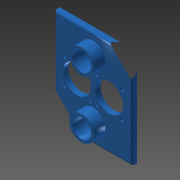
# Autodesk Inventor part: XCarriageV9Top
Saved by Autodesk Inventor 2015 (Build 190159000, 159)
## iProperties
Created: 2014-08-22
Part Number: XCarriageV9Top
Material: ABS Plastic
Document SubType Name: Modeling
Designer: Jack
Density: 1.06 g/cm^3
Appearance: Cyan
Author: Jack
Autodesk Inventor part; units mm, degrees
ref_plane "YZ Plane" through (0, 0, 0) normal (1, 0, 0) x (0, 1, 0)
ref_plane "XZ Plane" through (0, 0, 0) normal (0, 1, 0) x (-1, 0, 0)
ref_plane "XY Plane" through (0, 0, 0) normal (0, 0, 1) x (1, 0, 0)
sketch "Sketch1" plane through (0, 0, 0) normal (0, 1, 0) x (-1, 0, 0)
  line L0 (0, 0) -> (72, 0)
  line L1 (72, 0) -> (72, -90)
  line L2 (72, -90) -> (0, -90)
  line L3 (0, -90) -> (0, 0)
  dimension "d0" = 72
  dimension "d1" = 90
  constraints: 8 end point, 2 parallel, 1 horizontal, 1 perpendicular
  measures "d0" distance of L0.start L0.end
  measures "d1" distance of L2.end L0.start
extrude "Extrusion1" add sketch "Sketch1" along normal blind 5
sketch "Sketch2" plane through (0, 0, 0) normal (0, -1, 0) x (1, 0, 0)
  line L0 (-72, 0) -> (-72, -90) projected
  line L1 (-72, -90) -> (0, -90) projected
  circle A0 centre (-36, -72) radius 8.75
  circle A1 centre (-36, -18) radius 8.75
  circle A2 centre (-36, -18) radius 11.5
  circle A3 centre (-36, -72) radius 11.5
  dimension "d4" = 17.5
  dimension "d5" = 23
  dimension "d6" = 54
  dimension "d7" = 18
  dimension "d8" = 36
  constraints: 4 centre point, 2 coincident, 2 equal radius, 1 vertical alignment
  measures "d4" diameter of A1
  measures "d5" diameter of A2
  measures "d6" distance of A0.centre A1.centre
  measures "d7" distance from line of L1 A0.centre
  measures "d8" distance from line of L0 A0.centre
extrude "Extrusion2" add sketch "Sketch2" along normal blind 10.7
sketch "Sketch3" plane through (-36, 0, -18) normal (0, -1, 0) x (1, 0, 0)
  circle A0 centre (0, 0) radius 8.75 projected
  circle A1 centre (0, -54) radius 8.75 projected
  point P0 (36, 18)
extrude "Extrusion3" cut sketch "Sketch3" against normal up to surface (5 mm away)
sketch "Sketch4" plane through (0, 0, 0) normal (0, -1, 0) x (1, 0, 0)
  line L0 (0, 0) -> (-72, 0) projected
  line L1 (-72, 0) -> (-72, -90) projected
  line L2 (0, -90) -> (0, 0) projected
  circle A0 centre (-21, -45) radius 13
  circle A1 centre (-51, -45) radius 13
  dimension "d14" = 26
  dimension "d16" = 21
  dimension "d17" = 21
  dimension "d18" = 45
  constraints: 2 centre point, 1 equal radius, 1 horizontal alignment
  measures "d14" diameter of A1
  measures "d16" distance from line of L1 A1.centre
  measures "d17" distance from line of L2 A0.centre
  measures "d18" distance from line of L0 A0.centre
extrude "Extrusion4" cut sketch "Sketch4" against normal up to surface (5 mm away)
sketch "Sketch5" plane through (0, 0, 0) normal (0, -1, 0) x (1, 0, 0)
  circle A0 centre (-21, -45) radius 13 projected
  circle A1 centre (-51, -45) radius 13 projected
  circle A2 centre (-9, -57) radius 1.5
  circle A3 centre (-9, -33) radius 1.5
  circle A4 centre (-33, -57) radius 1.5
  circle A5 centre (-33, -33) radius 1.5
  circle A6 centre (-39, -33) radius 1.5
  circle A7 centre (-39, -57) radius 1.5
  circle A8 centre (-63, -57) radius 1.5
  circle A9 centre (-63, -33) radius 1.5
  dimension "d21" = 3
  dimension "d22" = 24
  dimension "d23" = 24
  dimension "d24" = 24
  dimension "d25" = 12
  dimension "d26" = 12
  dimension "d27" = 12
  constraints: 8 centre point, 7 equal radius, 6 horizontal alignment, 4 vertical alignment
  measures "d21" diameter of A2
  measures "d22" distance of A8.centre A7.centre
  measures "d23" distance of A2.centre A4.centre
  measures "d24" distance of A2.centre A3.centre
  measures "d25" horizontal distance of A0.centre A2.centre
  measures "d26" horizontal distance of A0.centre A2.centre
  measures "d27" horizontal distance of A1.centre A7.centre
extrude "Extrusion5" cut sketch "Sketch5" against normal up to surface (5 mm away) contours A2 | A3 | A4 | A5 | A6 | A7 | A8 | A9
sketch "Sketch6" plane through (0, 5, 0) normal (0, 1, 0) x (1, 0, 0)
  circle A0 centre (-39, 57) radius 1.5 projected
  circle A1 centre (-33, 33) radius 1.5 projected
  circle A2 centre (-33, 57) radius 1.5 projected
  circle A3 centre (-39, 33) radius 1.5 projected
  line L0 (-39, 60.1754) -> (-36.25, 58.5877)
  line L1 (-36.25, 58.5877) -> (-36.25, 55.4123)
  line L2 (-36.25, 55.4123) -> (-39, 53.8246)
  line L3 (-39, 53.8246) -> (-41.75, 55.4123)
  line L4 (-41.75, 55.4123) -> (-41.75, 58.5877)
  line L5 (-41.75, 58.5877) -> (-39, 60.1754)
  line L6 (-39, 36.1754) -> (-36.25, 34.5877)
  line L7 (-36.25, 34.5877) -> (-36.25, 31.4123)
  line L8 (-36.25, 31.4123) -> (-39, 29.8246)
  line L9 (-39, 29.8246) -> (-41.75, 31.4123)
  line L10 (-41.75, 31.4123) -> (-41.75, 34.5877)
  line L11 (-41.75, 34.5877) -> (-39, 36.1754)
  line L12 (-33, 36.1754) -> (-30.25, 34.5877)
  line L13 (-30.25, 34.5877) -> (-30.25, 31.4123)
  line L14 (-30.25, 31.4123) -> (-33, 29.8246)
  line L15 (-33, 29.8246) -> (-35.75, 31.4123)
  line L16 (-35.75, 31.4123) -> (-35.75, 34.5877)
  line L17 (-35.75, 34.5877) -> (-33, 36.1754)
  line L18 (-33, 60.1754) -> (-30.25, 58.5877)
  line L19 (-30.25, 58.5877) -> (-30.25, 55.4123)
  line L20 (-30.25, 55.4123) -> (-33, 53.8246)
  line L21 (-33, 53.8246) -> (-35.75, 55.4123)
  line L22 (-35.75, 55.4123) -> (-35.75, 58.5877)
  line L23 (-35.75, 58.5877) -> (-33, 60.1754)
  dimension "d30" = 5.5
  constraints: 48 end point, 4 coincident, 4 vertical, 3 equal length, 52 other
  measures "d30" distance between parallel lines of L1 L4
extrude "Extrusion6" cut sketch "Sketch6" against normal blind 2.5
fillet "Fillet1" radius 2 4 edges at (0, 0, -45) (-36, 0, -90) (-72, 0, -45) (-36, 0, 0)
fillet "Fillet2" radius 2 8 edges at (-0.5858, 0.5858, -89.4142) (0, 3.5, -90) (-0.5858, 0.5858, -0.5858) (0, 3.5, 0) (-71.4142, 0.5858, -0.5858) (-72, 3.5, 0) (-71.4142, 0.5858, -89.4142) (-72, 3.5, -90)
body "Solid1"
